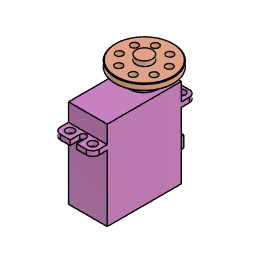
2024.10.14.Gripper_ver2 v11 (Autodesk Fusion 360 archive; units mm, degrees)
design "sts3032"
Autodesk Fusion 360 part; units mm, degrees
sketch "스케치1" plane through (0, 0, 0) normal (0, 0, 1) x (1, 0, 0)
  line L0 (6, 11.5) -> (-6, 11.5)
  line L1 (-6, 11.5) -> (-6, -11.5)
  line L2 (-6, -11.5) -> (6, -11.5)
  line L3 (6, -11.5) -> (6, 11.5)
  line L4 (6, 11.5) -> (-6, -11.5) construction
  line L5 (-6, 11.5) -> (6, -11.5) construction
  dimension "d1" = 12
  dimension "d2" = 23
  constraint horizontal L0
  constraint perpendicular L0 L1
  constraint parallel L0 L2
  constraint parallel L1 L3
  constraint coincident L4 origin
  constraint coincident L5 origin
  measures "d1" distance of L1.end L2.end
  measures "d2" distance of L0.end L1.end
extrude "돌출1" add sketch "스케치1" along normal blind 7 makes body 1
sketch "스케치2" plane through (0, 0, 0) normal (0, 0, -1) x (1, 0, 0)
  line L0 (6, -11.5) -> (6, 11.5)
  line L1 (6, 11.5) -> (-6, 11.5)
  line L2 (-6, 11.5) -> (-6, -11.5)
  line L3 (-6, -11.5) -> (6, -11.5)
extrude "돌출2" add sketch "스케치2" along normal blind 20.5 bodies 1
sketch "스케치3" plane through (0, 0, 0) normal (0, 0, 1) x (1, 0, 0)
  line L0 (-6, -16) -> (6, -16)
  line L1 (6, -16) -> (6, 16)
  line L2 (6, 16) -> (-6, 16)
  line L3 (-6, 16) -> (-6, -16)
  line L4 (-6, -16) -> (6, 16) construction
  line L5 (6, -16) -> (-6, 16) construction
  dimension "d7" = 12
  dimension "d8" = 32
  constraint horizontal L0
  constraint perpendicular L0 L1
  constraint parallel L0 L2
  constraint parallel L1 L3
  constraint coincident L4 origin
  constraint coincident L5 origin
  measures "d7" distance of L1.end L2.end
  measures "d8" distance of L0.end L1.end
extrude "돌출3" add sketch "스케치3" along normal blind 1.5 bodies 1
sketch "스케치4" plane through (0, 0, 7) normal (0, 0, 1) x (-1, 0, 0)
  line L0 (-6, 11.5) -> (-6, -11.5)
  line L1 (-6, -11.5) -> (6, -11.5)
  line L2 (6, -11.5) -> (6, 11.5)
  line L3 (6, 11.5) -> (-6, 11.5)
  circle A0 centre (0, -5.79) radius 4.5
  dimension "d11" = 9
  dimension "d12" = 5.71
  measures "d11" diameter of A0
  measures "d12" distance of L1 A0.centre
extrude "돌출4" add sketch "스케치4" along normal blind 1 contours A0 bodies 1
fillet "필렛1" radius 2 4 edges at (6, 16, 0.75) (-6, 16, 0.75) (6, -16, 0.75) (-6, -16, 0.75) on bodies 1
sketch "스케치5" plane through (0, 0, 1.5) normal (0, 0, 1) x (-1, 0, 0)
  arc A0 (4, -16) -> (6, -14) centre (4, -14) ccw
  line L0 (6, -14) -> (6, -11.5)
  line L1 (6, -11.5) -> (-6, -11.5)
  line L2 (-6, -11.5) -> (-6, -14)
  arc A1 (-6, -14) -> (-4, -16) centre (-4, -14) ccw
  line L3 (-4, -16) -> (4, -16)
  circle A2 centre (3.5, -14) radius 1.25
  circle A3 centre (-3.5, -14) radius 1.25
  line L4 (-6, -11.5) -> (6, -11.5)
  line L5 (1, -16) -> (-1, -16)
  line L6 (-1, -16) -> (-1, -13)
  line L7 (1, -13) -> (1, -16)
  line L8 (1, -16) -> (-1, -13) construction
  line L9 (-1, -16) -> (1, -13) construction
  circle A4 centre (0, -13) radius 1
  point P0 (0, -14.5)
  dimension "d17" = 2.5
  dimension "d18" = 2.5
  dimension "d19" = 2.5
  dimension "d20" = 2.5
  dimension "d21" = 2.5
  dimension "d22" = 2.5
  dimension "d23" = 2
  dimension "d24" = 3
  constraint horizontal L5
  constraint perpendicular L5 L6
  constraint parallel L6 L7
  constraint coincident L8 P0
  constraint coincident L9 P0
  constraint coincident L6.end A4
  measures "d17" diameter of A2
  measures "d18" diameter of A3
  measures "d19" distance of A2.centre L4
  measures "d20" distance of A3.centre L4
  measures "d21" distance of L0 A2.centre
  measures "d22" distance of L2 A3.centre
  measures "d23" distance of L6.end L7.start
  measures "d24" distance of L5.end L6.end
extrude "돌출5" cut sketch "스케치5" against normal blind 1.5 contours L3 L5 L6 L7 A4 | A4 | A2 | A3 bodies 1
sketch "스케치6" plane through (0, 0, 1.5) normal (0, 0, 1) x (-1, 0, 0)
  arc A0 (6, 14) -> (4, 16) centre (4, 14) ccw
  line L0 (4, 16) -> (-4, 16)
  arc A1 (-4, 16) -> (-6, 14) centre (-4, 14) ccw
  line L1 (-6, 14) -> (-6, 11.5)
  line L2 (-6, 11.5) -> (6, 11.5)
  line L3 (6, 11.5) -> (6, 14)
  circle A2 centre (3.5, 13.5) radius 1.25
  circle A3 centre (-3.5, 13.5) radius 1.25
  line L4 (1, 16) -> (-1, 16)
  line L5 (-1, 16) -> (-1, 13)
  line L6 (-1, 13) -> (1, 13)
  line L7 (1, 13) -> (1, 16)
  line L8 (1, 16) -> (-1, 13) construction
  line L9 (-1, 16) -> (1, 13) construction
  circle A4 centre (0, 13) radius 1
  point P0 (0, 14.5)
  dimension "d27" = 2.5
  dimension "d28" = 2.5
  dimension "d29" = 2.5
  dimension "d30" = 2.5
  dimension "d31" = 2.5
  dimension "d32" = 2.5
  dimension "d33" = 2
  dimension "d34" = 3
  constraint horizontal L4
  constraint perpendicular L4 L5
  constraint parallel L4 L6
  constraint parallel L5 L7
  constraint coincident L8 P0
  constraint coincident L9 P0
  constraint midpoint L6 A4.centre
  constraint coincident L5.end A4
  measures "d27" diameter of A2
  measures "d28" diameter of A3
  measures "d29" distance of L1 A3.centre
  measures "d30" distance of L3 A2.centre
  measures "d31" distance of L0 A2.centre
  measures "d32" distance of L0 A3.centre
  measures "d33" distance of L5.end L6.end
  measures "d34" distance of L4.end L5.end
extrude "돌출6" cut sketch "스케치6" against normal blind 1.5 contours L0 L4 L5 L7 A4 | L6 A4 | L6 A4 | A2 | A3 bodies 1
sketch "스케치7" plane through (0, 0, 8) normal (0, 0, 1) x (-1, 0, 0)
  circle A0 centre (0, -5.79) radius 4.5
sketch "스케치8" plane through (0, 0, 8) normal (0, 0, 1) x (-1, 0, 0)
  circle A0 centre (0, -6) radius 2
  dimension "d37" = 4
  measures "d37" diameter of A0
extrude "돌출7" add sketch "스케치8" along normal blind 2.5 bodies 1
sketch "스케치9" plane through (0, 0, 10.5) normal (0, 0, 1) x (-1, 0, 0)
  circle A0 centre (0, -6) radius 2
  circle A1 centre (0, -6) radius 3.5
  dimension "d40" = 7
  constraint concentric A0 A1
  measures "d40" diameter of A1
extrude "돌출8" add sketch "스케치9" against normal blind 2.5 bodies 1
chamfer "챔퍼2" distance 0.1 angle 45 1 edges at (4.1955, 7.4173, 8) on bodies 1
sketch "스케치13" plane through (0, 11.5, 0) normal (0, 1, 0) x (-1, 0, 0)
  line L0 (6, 0) -> (-6, 0)
  line L1 (-6, 0) -> (-6, -20.5)
  line L2 (-6, -20.5) -> (6, -20.5)
  line L3 (6, -20.5) -> (6, 0)
  line L4 (2.75, -11) -> (-2.75, -11)
  line L5 (-2.75, -11) -> (-2.75, -14.5)
  line L6 (-2.75, -14.5) -> (2.75, -14.5)
  line L7 (2.75, -14.5) -> (2.75, -11)
  line L8 (2.75, -11) -> (-2.75, -14.5) construction
  line L9 (-2.75, -11) -> (2.75, -14.5) construction
  point P0 (0, -12.75)
  dimension "d66" = 5.5
  dimension "d67" = 3.5
  dimension "d68" = 9.5
  dimension "d69" = 3.25
  constraint horizontal L4
  constraint perpendicular L4 L5
  constraint parallel L4 L6
  constraint parallel L5 L7
  constraint coincident L8 P0
  constraint coincident L9 P0
  measures "d66" distance of L5.end L6.end
  measures "d67" distance of L4.end L5.end
  measures "d68" distance of L2 L4
  measures "d69" distance of L3 L7
extrude "돌출12" add sketch "스케치13" along normal blind 4 contours L4 L5 L6 L7 bodies 1
sketch "스케치14" plane through (0, 0, 0) normal (0, 0, 1) x (1, 0, 0)
  circle A0 centre (35, 0) radius 9
  dimension "d72" = 18
  measures "d72" diameter of A0
extrude "돌출13" add sketch "스케치14" along normal blind 2 separate body makes body 2
copy_body "본체->구성요소1" bodies 2 removing the originals makes body 3 in component "Horn"
sketch "스케치15" plane through (0, 0, 0) normal (0, 0, 1) x (1, 0, 0)
sketch "스케치16" plane through (0, 0, 2) normal (0, 0, 1) x (-1, 0, 0)
  circle A0 centre (-35, 0) radius 9
  circle A1 centre (-35, 0) radius 6
  circle A2 centre (-29, 0) radius 1.1
  circle A3 centre (-35, 6) radius 1.1
  circle A4 centre (-35, -6) radius 1.1
  circle A5 centre (-41, 0) radius 1.1
  circle A6 centre (-39.2426, 4.2426) radius 1.1
  circle A7 centre (-30.7574, -4.2426) radius 1.1
  line L0 (-35, 0) -> (-41.0673, -6.0673)
  line L1 (-35, 0) -> (-26.4196, 0) construction
  circle A8 centre (-39.2426, -4.2426) radius 1.1
  line L2 (-35, 0) -> (-42, 7)
  line L3 (-35, 0) -> (-25.1005, 0) construction
  line L4 (-35, 0) -> (-25.88, 9.12)
  line L5 (-35, 0) -> (-22.1024, 0) construction
  circle A9 centre (-30.7574, 4.2426) radius 1.1
  line L6 (-35, 0) -> (-26.5147, -8.4853)
  line L7 (-35, 0) -> (-23.0742, 0) construction
  dimension "d75" = 12
  dimension "d76" = 2.2
  dimension "d77" = 2.2
  dimension "d78" = 2.2
  dimension "d79" = 2.2
  dimension "d80" = 2.2
  dimension "d81" = 2.2
  dimension "d82" = 135
  dimension "d83" = 2.2
  dimension "d84" = 135
  dimension "d85" = 45
  dimension "d86" = 2.2
  dimension "d87" = 45
  constraint concentric A0 A1
  constraint coincident A1 A2.centre
  constraint coincident A1 A3.centre
  constraint coincident A1 A4.centre
  constraint coincident A1 A5.centre
  constraint coincident A1 A6.centre
  constraint coincident A1 A7.centre
  constraint horizontal L1
  constraint coincident A0.centre A1.centre
  constraint coincident A1 A8.centre
  constraint coincident L0 A8.centre
  constraint horizontal L3
  constraint horizontal L5
  constraint coincident A1 A9.centre
  constraint coincident L4 A9.centre
  constraint horizontal L7
  constraint midpoint A7.centre L6
  measures "d75" diameter of A1
  measures "d76" diameter of A2
  measures "d77" diameter of A3
  measures "d78" diameter of A4
  measures "d79" diameter of A5
  measures "d80" diameter of A6
  measures "d81" diameter of A7
  measures "d82" angle of L0 L1
  measures "d83" diameter of A8
  measures "d84" angle of L2 L3
  measures "d85" angle of L4 L5
  measures "d86" diameter of A9
  measures "d87" angle of L6 L7
extrude "돌출1'" cut sketch "스케치16" against normal blind 2 contours A1 L4 A9 | A1 L4 A9 | A1 A7 L6 | A1 A7 L6 | A1 A6 L2 | A1 A6 L2 | A1 L4 A9 | A1 L4 A9 | A1 A7 L6 | A1 A7 L6 | A1 A6 L2 | A1 A6 L2 | A1 A3 | A1 A3 | A1 A4 | A1 A4 | A1 A5 | A1 A5 | A1 A2 | A1 A2 | A1 L0 A8 | A1 L0 A8 | A1 L0 A8 | A1 L0 A8 bodies 3 in component "Horn"
chamfer "챔퍼1" distance 0.2 angle 45 2 edges at (26.6091, -3.2545, 0) (26.6091, -3.2545, 2) on bodies 3 in component "Horn"
sketch "스케치17" plane through (0, 0, 2) normal (0, 0, 1) x (-1, 0, 0)
  circle A0 centre (-35, -6) radius 1.1
  circle A1 centre (-39.2426, 4.2426) radius 1.1
  circle A2 centre (-35, 6) radius 1.1
  circle A3 centre (-41, 0) radius 1.1
  circle A4 centre (-30.7574, -4.2426) radius 1.1
  circle A5 centre (-29, 0) radius 1.1
  circle A6 centre (-30.7574, 4.2426) radius 1.1
  circle A7 centre (-39.2426, -4.2426) radius 1.1
  circle A8 centre (-35, 0) radius 8.8
  circle A9 centre (-35, 0) radius 2.5
  dimension "d91" = 5
  constraint concentric A8 A9
  measures "d91" diameter of A9
extrude "돌출2'" add sketch "스케치17" along normal blind 1.5 contours A9 bodies 3 in component "Horn"
component "Horn" placed x (-1, 0, 0) y (0, -1, 0) z (0, 0, 1) at (35, 6, 10.5)
